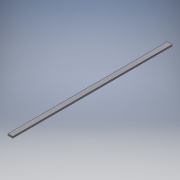
# Autodesk Inventor part: Rain T Slot
Saved by Autodesk Inventor 2019 (Build 230136000, 136)
## iProperties
Created: 2020-03-16
Part Number: Rain T Slot
Material: Generic
Document SubType Name: Modeling
Designer: Vijay
Density: 1 g/cm^3
Appearance: Default
Author: Vijay
Autodesk Inventor part; units mm, degrees
ref_plane "YZ Plane" through (0, 0, 0) normal (1, 0, 0) x (0, 1, 0)
ref_plane "XZ Plane" through (0, 0, 0) normal (0, 1, 0) x (-1, 0, 0)
ref_plane "XY Plane" through (0, 0, 0) normal (0, 0, 1) x (1, 0, 0)
sketch "Sketch1" plane through (0, 0, 0) normal (0, 0, 1) x (1, 0, 0)
  line L0 (8.25, 13) -> (8.25, 9.6642) projected
  line L1 (8.25, 9.6642) -> (4.1, 5.5142) projected
  line L2 (4.1, 5.5142) -> (-4.1, 5.5142) projected
  line L3 (-4.1, 5.5142) -> (-8.25, 9.6642) projected
  line L4 (-8.25, 9.6642) -> (-8.25, 13) projected
  line L5 (-8.25, 13) -> (-4.1, 13) projected
  line L6 (-4.1, 13) -> (-4.1, 14) projected
  line L7 (-4.1, 14) -> (-5.1, 14) projected
  line L8 (-5.1, 14) -> (-5.1, 15) projected
  line L9 (-5.1, 15) -> (-13, 15) projected
  arc A0 (-13, 15) -> (-15, 13) centre (-13, 13) ccw projected
  line L10 (-15, 13) -> (-15, 5.1) projected
  line L11 (-15, 5.1) -> (-14, 5.1) projected
  line L12 (-14, 5.1) -> (-14, 4.1) projected
  line L13 (-14, 4.1) -> (-13, 4.1) projected
  line L14 (-13, 4.1) -> (-13, 8.25) projected
  line L15 (-13, 8.25) -> (-9.6642, 8.25) projected
  line L16 (-9.6642, 8.25) -> (-5.5142, 4.1) projected
  line L17 (-5.5142, 4.1) -> (-5.5142, -4.1) projected
  line L18 (-5.5142, -4.1) -> (-9.6642, -8.25) projected
  line L19 (-9.6642, -8.25) -> (-13, -8.25) projected
  line L20 (-13, -8.25) -> (-13, -4.1) projected
  line L21 (-13, -4.1) -> (-14, -4.1) projected
  line L22 (-14, -4.1) -> (-14, -5.1) projected
  line L23 (-14, -5.1) -> (-15, -5.1) projected
  line L24 (-15, -5.1) -> (-15, -13) projected
  arc A1 (-15, -13) -> (-13, -15) centre (-13, -13) ccw projected
  line L25 (-13, -15) -> (-5.1, -15) projected
  line L26 (-5.1, -15) -> (-5.1, -14) projected
  line L27 (-5.1, -14) -> (-4.1, -14) projected
  line L28 (-4.1, -14) -> (-4.1, -13) projected
  line L29 (-4.1, -13) -> (-8.25, -13) projected
  line L30 (-8.25, -13) -> (-8.25, -9.6642) projected
  line L31 (-8.25, -9.6642) -> (-4.1, -5.5142) projected
  line L32 (-4.1, -5.5142) -> (4.1, -5.5142) projected
  line L33 (4.1, -5.5142) -> (8.25, -9.6642) projected
  line L34 (8.25, -9.6642) -> (8.25, -13) projected
  line L35 (8.25, -13) -> (4.1, -13) projected
  line L36 (4.1, -13) -> (4.1, -14) projected
  line L37 (4.1, -14) -> (5.1, -14) projected
  line L38 (5.1, -14) -> (5.1, -15) projected
  line L39 (5.1, -15) -> (13, -15) projected
  arc A2 (13, -15) -> (15, -13) centre (13, -13) ccw projected
  line L40 (15, -13) -> (15, -5.1) projected
  line L41 (15, -5.1) -> (14, -5.1) projected
  line L42 (14, -5.1) -> (14, -4.1) projected
  line L43 (14, -4.1) -> (13, -4.1) projected
  line L44 (13, -4.1) -> (13, -8.25) projected
  line L45 (13, -8.25) -> (9.6642, -8.25) projected
  line L46 (9.6642, -8.25) -> (5.5142, -4.1) projected
  line L47 (5.5142, -4.1) -> (5.5142, 4.1) projected
  line L48 (5.5142, 4.1) -> (9.6642, 8.25) projected
  line L49 (9.6642, 8.25) -> (13, 8.25) projected
  line L50 (13, 8.25) -> (13, 4.1) projected
  line L51 (13, 4.1) -> (14, 4.1) projected
  line L52 (14, 4.1) -> (14, 5.1) projected
  line L53 (14, 5.1) -> (15, 5.1) projected
  line L54 (15, 5.1) -> (15, 13) projected
  arc A3 (15, 13) -> (13, 15) centre (13, 13) ccw projected
  line L55 (13, 15) -> (5.1, 15) projected
  line L56 (5.1, 15) -> (5.1, 14) projected
  line L57 (5.1, 14) -> (4.1, 14) projected
  line L58 (4.1, 14) -> (4.1, 13) projected
  line L59 (4.1, 13) -> (8.25, 13) projected
  arc A4 (9.75, -12.5) -> (10.75, -13.5) centre (10.75, -12.5) ccw projected
  line L60 (9.75, -12.5) -> (9.75, -10.75) projected
  arc A5 (10.75, -9.75) -> (9.75, -10.75) centre (10.75, -10.75) ccw projected
  line L61 (10.75, -9.75) -> (12.5, -9.75) projected
  arc A6 (13.5, -10.75) -> (12.5, -9.75) centre (12.5, -10.75) ccw projected
  line L62 (13.5, -10.75) -> (13.5, -12.5) projected
  arc A7 (12.5, -13.5) -> (13.5, -12.5) centre (12.5, -12.5) ccw projected
  line L63 (12.5, -13.5) -> (10.75, -13.5) projected
  arc A8 (-13.5, 10.75) -> (-12.5, 9.75) centre (-12.5, 10.75) ccw projected
  line L64 (-13.5, 10.75) -> (-13.5, 12.5) projected
  arc A9 (-12.5, 13.5) -> (-13.5, 12.5) centre (-12.5, 12.5) ccw projected
  line L65 (-12.5, 13.5) -> (-10.75, 13.5) projected
  arc A10 (-9.75, 12.5) -> (-10.75, 13.5) centre (-10.75, 12.5) ccw projected
  line L66 (-9.75, 12.5) -> (-9.75, 10.75) projected
  arc A11 (-10.75, 9.75) -> (-9.75, 10.75) centre (-10.75, 10.75) ccw projected
  line L67 (-10.75, 9.75) -> (-12.5, 9.75) projected
  circle A12 centre (0, 0) radius 3.4 projected
  line L68 (9.75, 10.75) -> (9.75, 12.5) projected
  arc A13 (10.75, 13.5) -> (9.75, 12.5) centre (10.75, 12.5) ccw projected
  line L69 (10.75, 13.5) -> (12.5, 13.5) projected
  arc A14 (13.5, 12.5) -> (12.5, 13.5) centre (12.5, 12.5) ccw projected
  line L70 (13.5, 12.5) -> (13.5, 10.75) projected
  arc A15 (12.5, 9.75) -> (13.5, 10.75) centre (12.5, 10.75) ccw projected
  line L71 (12.5, 9.75) -> (10.75, 9.75) projected
  arc A16 (9.75, 10.75) -> (10.75, 9.75) centre (10.75, 10.75) ccw projected
  arc A17 (-12.5, -9.75) -> (-13.5, -10.75) centre (-12.5, -10.75) ccw projected
  line L72 (-12.5, -9.75) -> (-10.75, -9.75) projected
  arc A18 (-9.75, -10.75) -> (-10.75, -9.75) centre (-10.75, -10.75) ccw projected
  line L73 (-9.75, -10.75) -> (-9.75, -12.5) projected
  arc A19 (-10.75, -13.5) -> (-9.75, -12.5) centre (-10.75, -12.5) ccw projected
  line L74 (-10.75, -13.5) -> (-12.5, -13.5) projected
  arc A20 (-13.5, -12.5) -> (-12.5, -13.5) centre (-12.5, -12.5) ccw projected
  line L75 (-13.5, -12.5) -> (-13.5, -10.75) projected
  line L76 (-6, -13) -> (6, -13)
  line L77 (6, -13) -> (6, -9)
  line L78 (6, -9) -> (-6, -9)
  line L79 (-6, -9) -> (-6, -13)
  line L80 (0, -5.5142) -> (0, -26.3036) construction
  point P0 (0, 0)
  dimension "d0" = 4
  dimension "d1" = 12
  constraints: 10 end point, 2 parallel, 1 collinear, 1 horizontal, 1 midpoint, 1 perpendicular, 1 vertical, 1 other
  measures "d0" distance between parallel lines of L76 L78
  measures "d1" distance of L76.start L76.end
extrude "Extrusion1" add sketch "Sketch1" against normal blind 400 contours L76 L29 L79 L78 L77 L35
sketch "Sketch2" plane through (-6, -13, 0) normal (0, -1, 0) x (1, 0, 0)
  circle A0 centre (6.0003, -10) radius 3 projected
  circle A1 centre (6.0003, -35) radius 3 projected
  circle A2 centre (6.0003, -10) radius 1.25
  point P0 (6, 0)
  dimension "d4" = 2.5
  constraints: 1 centre point, 1 coincident
  measures "d4" diameter of A2
extrude "Extrusion2" cut sketch "Sketch2" against normal blind 400 contours A2
pattern_linear "Rectangular Pattern1" count 8 spacing 50 along (0, 0, -1) of "Extrusion2"
body "Solid1"
